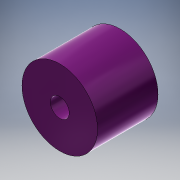
# Autodesk Inventor part: housing_legs
Saved by Autodesk Inventor 2017 (Build 210142000, 142)
## iProperties
Created: 2017-09-14
Part Number: housing_legs
Material: Ogólny
Document SubType Name: Modeling
Designer: Speed King
Density: 1 g/cm^3
Appearance: Gładki - fioletowy
Author: Speed King
Autodesk Inventor part; units mm, degrees
ref_plane "YZ Plane" through (0, 0, 0) normal (1, 0, 0) x (0, 1, 0)
ref_plane "XZ Plane" through (0, 0, 0) normal (0, 1, 0) x (-1, 0, 0)
ref_plane "XY Plane" through (0, 0, 0) normal (0, 0, 1) x (1, 0, 0)
sketch "Szkic1" plane through (0, 0, 0) normal (0, 1, 0) x (-1, 0, 0)
  circle A0 centre (0, 0) radius 5
  dimension "d0" = 10
  constraints: 1 centre point, 1 coincident
  measures "d0" diameter of A0
extrude "Wyciągnięcie proste1" add sketch "Szkic1" along normal blind 8
sketch "Szkic2" plane through (0, 8, 0) normal (0, 1, 0) x (1, 0, 0)
  line L0 (-2.75, -1.5877) -> (-2.75, 1.5877)
  line L1 (-2.75, 1.5877) -> (0, 3.1754)
  line L2 (0, 3.1754) -> (2.75, 1.5877)
  line L3 (2.75, 1.5877) -> (2.75, -1.5877)
  line L4 (2.75, -1.5877) -> (0, -3.1754)
  line L5 (0, -3.1754) -> (-2.75, -1.5877)
  line L6 (0, 7) -> (0, -7) projected
  point P0 (0, 0)
  point P1 (0, 0)
  dimension "d3" = 5.5
  constraints: 12 end point, 1 coincident, 1 parallel, 13 other
  measures "d3" distance between parallel lines of L3 L0
extrude "Wyciągnięcie proste2" cut sketch "Szkic2" against normal blind 3
sketch "Szkic3" plane through (0, 5, 0) normal (0, 1, 0) x (1, 0, 0)
  circle A0 centre (0, 0) radius 5 projected
  circle A1 centre (0, 0) radius 1.25
  dimension "d6" = 2.5
  constraints: 1 centre point, 1 coincident
  measures "d6" diameter of A1
extrude "Wyciągnięcie proste3" cut sketch "Szkic3" against normal through all contours A1
